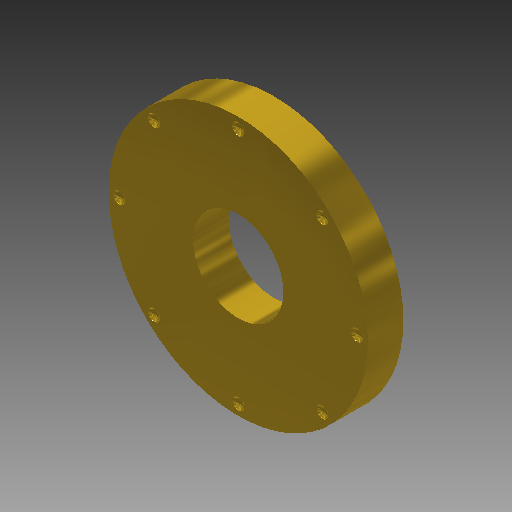
# Autodesk Inventor part: Plate between E2 and E3
Saved by Autodesk Inventor 2017 (Build 210142000, 142)
## iProperties
Created: 2009-05-07
Part Number: Plate between E2 and E3
Document SubType Name: Modeling
Designer: Serena
Material: Generic
Density: 1 g/cm^3
Appearance: Glossy - Gold
Author: Serena
Autodesk Inventor part; units mm, degrees
ref_plane "YZ Plane" through (0, 0, 0) normal (1, 0, 0) x (0, 1, 0)
ref_plane "XZ Plane" through (0, 0, 0) normal (0, 1, 0) x (-1, 0, 0)
ref_plane "XY Plane" through (0, 0, 0) normal (0, 0, 1) x (1, 0, 0)
sketch "Sketch1" plane through (0, 0, 0) normal (0, 0, 1) x (1, 0, 0)
  circle A0 centre (0, 0) radius 6.35
  circle A1 centre (0, 0) radius 18.25
  dimension "d0" = 12.7
  dimension "d1" = 36.5
  constraints: 2 centre point, 1 coincident
  measures "d0" diameter of A0
  measures "d1" diameter of A1
extrude "Extrusion1" add sketch "Sketch1" along normal blind 5
sketch "Sketch2" plane through (0, 0, 5) normal (0, 0, 1) x (1, 0, 0)
  circle A0 centre (0, 0) radius 6.35 projected
  circle A1 centre (0, 0) radius 18.25 projected
  circle A2 centre (0, 0) radius 7.1
  dimension "d4" = 14.2
  constraints: 1 centre point, 1 coincident
  measures "d4" diameter of A2
sketch "Sketch3" plane through (0, 0, 0) normal (0, 1, 0) x (-1, 0, 0)
  line L0 (6.35, 0) -> (6.35, 5) projected
  line L1 (18.25, 0) -> (18.25, 5) projected
  line L2 (-18.25, 5) -> (18.25, 5) projected
  line L3 (-18.25, 0) -> (18.25, 0) projected
  line L4 (7.85, 5) -> (7.85, 0)
  line L5 (16.75, 5) -> (16.75, 0)
  line L6 (16.75, 5) -> (16.75, 7)
  line L7 (7.85, 5) -> (7.85, 8)
  line L8 (7.85, 0) -> (7.85, -2)
  circle A0 centre (16.75, 5.5) radius 1
  line L9 (16.75, 5) -> (16.75, 4.5)
  line L10 (16.75, 5) -> (15.884, 5)
  line L11 (16.75, 5) -> (17.616, 5)
  arc A1 (15.884, 5) -> (16.75, 4.5) centre (16.75, 5.5) ccw
  arc A2 (16.75, 4.5) -> (17.616, 5) centre (16.75, 5.5) ccw
  dimension "d5" = 1.5
  dimension "d6" = 1.5
  dimension "d9" = 0.5
  dimension "d10" = 2
  constraints: 16 end point, 7 point on circle, 7 point on line, 4 concentric, 3 centre point, 2 collinear, 1 parallel
  measures "d5" distance between parallel lines of L1 L5
  measures "d6" distance between parallel lines of L0 L4
  measures "d9" distance of L5.start L9.end
  measures "d10" diameter of A0
revolve "Revolution1" cut sketch "Sketch3" angle 360 about axis through (-16.75, 0, 5) along (0, 0, -1) picked at (17.2864, 4.9436) contours L5 L2 A0
pattern_circular "Circular Pattern1" count 8 over 360 about axis through (0, 0, 0) along (0, 0, 1) of "Revolution1"
sketch "Sketch4" plane through (0, 0, 0) normal (0, 1, 0) x (-1, 0, 0)
  line L0 (18.25, 0) -> (18.25, 5) projected
  line L1 (6.35, 0) -> (6.35, 5) projected
  line L2 (-18.25, 0) -> (18.25, 0) projected
  line L3 (-18.25, 5) -> (18.25, 5) projected
  line L4 (7.85, 5) -> (7.85, 0)
  line L5 (7.85, 0) -> (7.85, -3)
  circle A0 centre (7.85, -0.5) radius 1
  line L6 (7.85, 0) -> (7.85, 0.5)
  line L7 (7.85, 0) -> (6.984, 0)
  line L8 (7.85, 0) -> (8.716, 0)
  arc A1 (8.716, 0) -> (7.85, 0.5) centre (7.85, -0.5) ccw
  arc A2 (7.85, 0.5) -> (6.984, 0) centre (7.85, -0.5) ccw
  dimension "d15" = 1.5
  dimension "d16" = 0.5
  dimension "d17" = 2
  constraints: 10 end point, 7 point on circle, 6 point on line, 3 centre point, 3 concentric, 1 collinear, 1 perpendicular
  measures "d15" distance between parallel lines of L1 L4
  measures "d16" distance of L4.end L6.end
  measures "d17" diameter of A0
revolve "Revolution2" cut sketch "Sketch4" angle 360 about axis through (-7.85, 0, 5) along (0, 0, -1) picked at (8.3864, 0.0564) contours L2 L4 A0
pattern_circular "Circular Pattern2" count 6 over 360 about axis through (0, 0, 0) along (0, 0, 1) of "Revolution2"
body "Solid1"
